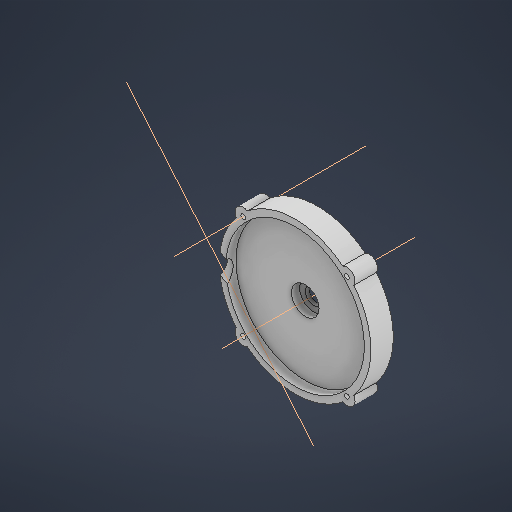
# Autodesk Inventor part: Case Part 2
Saved by Autodesk Inventor 2025.3 (Build 293356030, 356C)
## iProperties
Created: 2025-09-18
Part Number: Case Part 2
Material: Generic
Document SubType Name: Modeling
Designer: yo
Density: 1 g/cm^3
Appearance: Default
Author: yo
Autodesk Inventor part; units mm, degrees
ref_plane "YZ Plane" through (0, 0, 0) normal (1, 0, 0) x (0, 1, 0)
sketch "Sketch1" plane through (0, 0, 0) normal (0, 0, 1) x (1, 0, 0)
  circle A0 centre (0, 0) radius 5
  circle A1 centre (0, 0) radius 8.45
  circle A2 centre (0, 0) radius 42.5
  circle A3 centre (0, 0) radius 45 construction
  circle A4 centre (-31.8198, 31.8198) radius 1.45
  arc A5 (-28.0933, 35.1535) -> (-35.1535, 28.0933) centre (-31.8198, 31.8198) ccw
  arc A6 (-35.1535, -28.0933) -> (-28.0933, -35.1535) centre (-31.8198, -31.8198) ccw
  circle A7 centre (-31.8198, -31.8198) radius 1.45
  arc A8 (28.0933, -35.1535) -> (35.1535, -28.0933) centre (31.8198, -31.8198) ccw
  circle A9 centre (31.8198, -31.8198) radius 1.45
  arc A10 (35.1535, 28.0933) -> (28.0933, 35.1535) centre (31.8198, 31.8198) ccw
  circle A11 centre (31.8198, 31.8198) radius 1.45
  line L0 (-31.8198, 31.8198) -> (31.8198, 31.8198) construction
  arc A12 (29.278, 36.1255) -> (-29.278, 36.1255) centre (0, 0) ccw
  arc A13 (-36.1255, 29.278) -> (-36.1255, -29.278) centre (0, 0) ccw
  arc A14 (-29.278, -36.1255) -> (29.278, -36.1255) centre (0, 0) ccw
  arc A15 (36.1255, -29.278) -> (36.1255, 29.278) centre (0, 0) ccw
  point P0 (0, -46.5)
  point P1 (0, 46.5)
  dimension "d2" = 10
  dimension "d3" = 16.9
  dimension "d4" = 85
  dimension "d5" = 90
  dimension "d6" = 2.9
  dimension "d7" = 5
  dimension "d8" = 360
  dimension "d24" = 93
  constraints: 29 point on circle, 16 centre point, 10 coincident, 3 concentric, 2 end point, 1 horizontal, 25 other
  measures "d2" diameter of A0
  measures "d3" diameter of A1
  measures "d4" diameter of A2
  measures "d5" diameter of A3
  measures "d6" diameter of A4
  measures "d7" radius of A5
  measures "d24" distance of point (0, -46.5) point (0, 46.5)
extrude "Extrusion1" add sketch "Sketch1" against normal blind 3.75 contours A12 A10 A15 A8 A14 A6 A13 A5
extrude "Extrusion2" add sketch "Sketch1" along normal mid plane 7.5 contours A2
extrude "Extrusion3" add sketch "Sketch1" along normal blind 10 contours A12 A10 A15 A8 A14 A6 A13 A5
sketch "Sketch2" plane through (0, 0, 10) normal (0, 0, 1) x (1, 0, 0)
  arc A0 (-36.1255, 29.278) -> (-36.1255, -29.278) centre (0, 0) ccw projected
  line L0 (-46.5, 0) -> (-46.5, -31.8198) construction
  circle A1 centre (-31.8198, -31.8198) radius 1.45 projected
  constraints: 2 end point, 1 horizontal alignment, 1 point on circle, 1 tangent, 1 vertical
ref_plane "Work Plane1" through (-46.5, 0, 10) normal (-0.9659, 0, -0.2588) x (0, -1, 0)
sketch "Sketch3" plane through (-46.5, 0, 10) normal (-0.9659, 0, -0.2588) x (0, -1, 0)
  line L0 (0, 0) -> (31.8198, 0) projected
  line L1 (0, 0) -> (0, -21.6943) construction
  constraints: 2 end point, 1 vertical
ref_plane "Work Plane2" through (-46.5, 0, 10) normal (-0.8365, 0.5, -0.2241) x (0.2588, 0, -0.9659)
sketch "Sketch4" plane through (-46.5, 0, 10) normal (-0.8365, 0.5, -0.2241) x (0.2588, 0, -0.9659)
  circle A0 centre (0, 0) radius 5.325
  point P0 (21.6943, -21.1637)
  point P1 (0, 0)
  dimension "d20" = 10.65
  constraints: 1 centre point, 1 coincident
  measures "d20" diameter of A0
extrude "Extrusion5" cut sketch "Sketch4" along normal mid plane 20
sketch "Sketch5" plane through (0, 0, -3.75) normal (0, 0, -1) x (-1, 0, 0)
  circle A0 centre (0, 0) radius 5 projected
  circle A1 centre (0, 0) radius 8.45 projected
extrude "Extrusion6" add sketch "Sketch5" against normal blind 2.5
body "Solid1"
